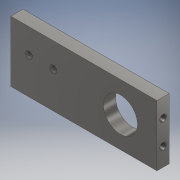
# Autodesk Inventor part: DriverElevatorConnection
Saved by Autodesk Inventor 2017 (Build 210142000, 142)
## iProperties
Created: 2016-12-12
Part Number: DriverElevatorConnection
Material: Steel, Carbon
Document SubType Name: Modeling
Designer: umr
Density: 7.85 g/cm^3
Appearance: Semi-Polished
Author: umr
Autodesk Inventor part; units mm, degrees
ref_plane "YZ Plane" through (0, 0, 0) normal (1, 0, 0) x (0, 1, 0)
ref_plane "XZ Plane" through (0, 0, 0) normal (0, 1, 0) x (-1, 0, 0)
ref_plane "XY Plane" through (0, 0, 0) normal (0, 0, 1) x (1, 0, 0)
sketch "Sketch1" plane through (0, 0, 0) normal (0, 1, 0) x (-1, 0, 0)
  line L0 (0, 0) -> (120, 0)
  line L1 (120, 0) -> (120, -50)
  line L2 (120, -50) -> (0, -50)
  line L3 (0, -50) -> (0, 0)
  circle A0 centre (30, -25) radius 14
  dimension "d0" = 120
  dimension "d1" = 50
  dimension "d4" = 28
  dimension "d5" = 30
  constraints: 8 end point, 2 parallel, 1 centre point, 1 horizontal, 1 perpendicular
  measures "d0" distance of L1.end L2.end
  measures "d1" distance of L0.end L1.end
  measures "d4" diameter of A0
  measures "d5" distance from line of L3 A0.centre
extrude "Extrusion2" add sketch "Sketch1" along normal blind 10
sketch "Sketch2" plane through (0, 10, 0) normal (0, 1, 0) x (1, 0, 0)
  circle A0 centre (-105, 20) radius 2.75
  line L0 (-120, 50) -> (-120, 0) projected
  line L1 (0, 50) -> (-120, 50) projected
  circle A1 centre (-85, 20) radius 2.75
  line L2 (-120, 0) -> (0, 0) projected
  dimension "d8" = 5.5
  dimension "d9" = 50
  dimension "d11" = 15
  dimension "d14" = 20
  dimension "d21" = 20
  constraints: 2 centre point, 1 horizontal, 2 other
  measures "d8" diameter of A0
  measures "d9" distance of L0.start L0.end
  measures "d11" distance from line of L0 A0.centre
  measures "d14" distance of A0.centre A1.centre
  measures "d21" distance from line of L2 A0.centre
extrude "Extrusion3" cut sketch "Sketch2" against normal blind 10
sketch "Sketch3" plane through (0, 0, 0) normal (1, 0, 0) x (0, 0, -1)
  circle A0 centre (15, 5) radius 2.75
  line L0 (0, 10) -> (50, 10) projected
  line L1 (0, 0) -> (0, 10) projected
  circle A1 centre (35, 5) radius 2.75
  dimension "d22" = 5.5
  dimension "d23" = 10
  dimension "d24" = 50
  dimension "d25" = 5
  dimension "d28" = 20
  dimension "d33" = 15
  constraints: 2 centre point, 1 horizontal, 2 other
  measures "d22" diameter of A0
  measures "d23" distance of L1.start L0.start
  measures "d24" distance of L0.start L0.end
  measures "d25" distance from line of L0 A0.centre
  measures "d28" distance of A0.centre A1.centre
  measures "d33" distance from line of L1 A0.centre
extrude "Extrusion4" cut sketch "Sketch3" against normal blind 5
equation "\"d25\" = 0.5 * d23"
equation "\"d33\" = -0.5 * d28 + 0.5 * d24"
body "Solid2"
